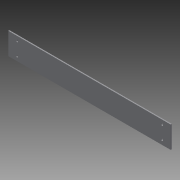
# Autodesk Inventor part: polycarb back
Saved by Autodesk Inventor 2015 SP1 (Build 190203100, 203)
## iProperties
Created: 2015-01-16
Part Number: polycarb back
Material: Generic
Document SubType Name: Modeling
Designer: Jarod
Density: 1 g/cm^3
Appearance: Default
Author: Jarod
Autodesk Inventor part; units mm, degrees
ref_plane "YZ Plane" through (0, 0, 0) normal (1, 0, 0) x (0, 1, 0)
ref_plane "XZ Plane" through (0, 0, 0) normal (0, 1, 0) x (-1, 0, 0)
ref_plane "XY Plane" through (0, 0, 0) normal (0, 0, 1) x (1, 0, 0)
sketch "Sketch1" plane through (0, 0, 0) normal (0, 0, 1) x (1, 0, 0)
  line L0 (0, 0) -> (469.9, 0)
  line L1 (469.9, 0) -> (469.9, 63.5)
  line L2 (469.9, 63.5) -> (0, 63.5)
  line L3 (0, 63.5) -> (0, 0)
  dimension "d0" = 469.9
  dimension "d1" = 63.5
  constraints: 8 end point, 2 parallel, 1 horizontal, 1 perpendicular
  measures "d0" distance of L2.end L1.end
  measures "d1" distance of L1.end L0.end
extrude "Extrusion1" add sketch "Sketch1" along normal blind 3.175
sketch "Sketch2" plane through (0, 0, 3.175) normal (0, 0, 1) x (1, 0, 0)
  line L0 (0, 0) -> (469.9, 0) projected
  line L1 (469.9, 0) -> (469.9, 63.5) projected
  line L2 (469.9, 63.5) -> (0, 63.5) projected
  line L3 (0, 63.5) -> (0, 0) projected
  point P0 (25.4, 50.8)
  point P1 (25.4, 12.7)
  point P2 (444.5, 12.7)
  point P3 (444.5, 50.8)
  dimension "d4" = 25.4
  dimension "d6" = 12.7
  dimension "d7" = 25.4
  dimension "d9" = 25.4
  dimension "d10" = 25.4
  dimension "d11" = 12.7
  dimension "d19" = 50.8
  dimension "d20" = 50.8
  measures "d4" distance from line of L3 point (25.4, 50.8)
  measures "d6" distance from line of L0 point (25.4, 12.7)
  measures "d7" distance from line of L3 point (25.4, 12.7)
  measures "d9" distance from line of L1 point (444.5, 50.8)
  measures "d10" distance from line of L1 point (444.5, 12.7)
  measures "d11" distance from line of L0 point (444.5, 12.7)
  measures "d19" distance from line of L0 point (444.5, 50.8)
  measures "d20" distance from line of L0 point (25.4, 50.8)
hole "Hole1" at (25.4, 50.8, 3.175) at (25.4, 12.7, 3.175) at (444.5, 12.7, 3.175) at (444.5, 50.8, 3.175) direction (0, 0, -1) diameter 6.35 end through all
body "Solid1"
